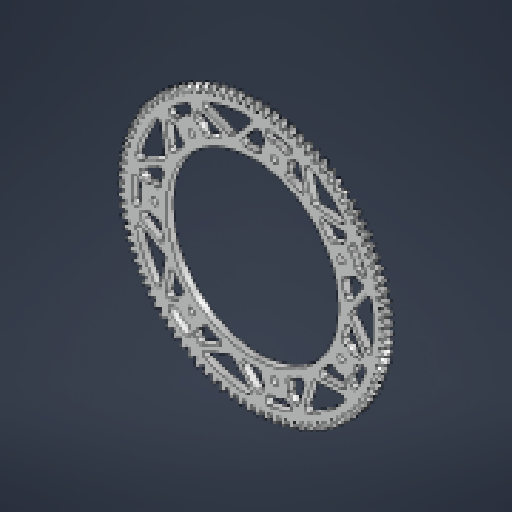
# Autodesk Inventor part: PLATE,TURRET,GEAR
Saved by Autodesk Inventor 2026 (Build 300175000, 175)
## iProperties
CustomPartVersion: 1
Created: 2026-02-09
Part Number: PLATE,TURRET,GEAR
Material: Aluminum 6061
Document SubType Name: Modeling
Designer: littl
Categories: <?xml version="1.0" encoding="UTF-16"?> <MemberInstance><Categories><FamilyTemplate><FamilyTemplateParameter ValueType="xs:double" Id="1" ObjectReferenceKey="da_z" ObjectType="kUserParameterObject"/><FamilyTemplateParameter ValueType="xs:double" Id="2" ObjectReferenceKey="da_b" ObjectType="kUserParameterObject"/><FamilyTemplateParameter ValueType="xs:double" Id="3" ObjectReferenceKey="da_beta" ObjectType="kUserParameterObject"/><FamilyTemplateParameter ValueType="xs:double" Id="4" ObjectReferenceKey="da_da" ObjectType="kUserParameterObject"/><FamilyTemplateParameter ValueType="xs:double" Id="5" ObjectReferenceKey="da_aw" ObjectType="kUserParameterObject"/><FamilyTemplateParameter ValueType="xs:string" Id="6" ObjectReferenceKey="EAIAABAAAAC/AAAAAAAAAIAAAAAAAAAA" ObjectType="83910656" SubObjectId="SurfaceGeometry"/></FamilyTemplate><ParamToTemplateMap><ParamToTemplate CategoryParameter="//CategoryParameter[@InternalName='046C89C9-8512-4d59-83FE-43B91F4F132A']" TemplateParameter="1"/><ParamToTemplate CategoryParameter="//CategoryParameter[@InternalName='2552DF32-E462-4b46-AEBF-C6C7768E72AC']" TemplateParameter="2"/><ParamToTemplate CategoryParameter="//CategoryParameter[@InternalName='C9EE641D-15FC-4fae-A226-E94C4372FDD7']" TemplateParameter="3"/><ParamToTemplate><ParamToTemplate CategoryParameter="//CategoryParameter[@InternalName='00B6519A-459B-49c7-AD84-2E56D39A5744']" ConstantValue="0.000000"/></ParamToTemplate><ParamToTemplate><ParamToTemplate CategoryParameter="//CategoryParameter[@InternalName='04B31F0E-C7A6-4894-AA32-9629BEFACF47']" ConstantValue="1.000000"/></ParamToTemplate><ParamToTemplate><ParamToTemplate CategoryParameter="//CategoryParameter[@InternalName='43CBEC2E-7847-49e7-A936-2F7889FCB2D9']" ConstantValue="0.250000"/></ParamToTemplate><ParamToTemplate><ParamToTemplate CategoryParameter="//CategoryParameter[@InternalName='B1EFC894-105D-4ebd-86BF-FA20ED196853']" ConstantValue="0.350000"/></ParamToTemplate><ParamToTemplate><ParamToTemplate CategoryParameter="//CategoryParameter[@InternalName='51175063-3D10-4879-93E8-6246FE8B403D']" ConstantValue="2061532430.657340"/></ParamToTemplate><ParamToTemplate><ParamToTemplate CategoryParameter="//CategoryParameter[@InternalName='A3A52E27-4454-46a9-B0BD-C932399B70AF']" ConstantValue="0.300000"/></ParamToTemplate><ParamToTemplate><ParamToTemplate CategoryParameter="//CategoryParameter[@InternalName='91B76062-C214-41d9-B1B9-14D2AB99603D']" ConstantValue="0.254000"/></ParamToTemplate><ParamToTemplate><ParamToTemplate CategoryParameter="//CategoryParameter[@InternalName='374E806E-8B8A-4dda-A9AA-1039D6500AD2']" ConstantValue="3.937008"/></ParamToTemplate><ParamToTemplate><ParamToTemplate CategoryParameter="//CategoryParameter[@InternalName='2D373A89-B862-43d6-8D0B-0CBF12AB9F6C']" ConstantValue="0.349066"/></ParamToTemplate><ParamToTemplate CategoryParameter="//CategoryParameter[@InternalName='37777632-D6A2-4fac-9D53-DB8ACD95C989']" TemplateParameter="4"/><ParamToTemplate CategoryParameter="//CategoryParameter[@InternalName='FD1017F1-B727-4f7e-9707-0F86F1FF9423']" TemplateParameter="5"/><ParamToTemplate><ParamToTemplate CategoryParameter="//CategoryParameter[@InternalName='9E1B4470-B2D3-4ff1-B813-535BB4CDF51A']" ConstantValue="3523220.976809"/></ParamToTemplate><ParamToTemplate><ParamToTemplate CategoryParameter="//CategoryParameter[@InternalName='F8452263-BFF6-458c-9FB1-07C4B99E95CD']" ConstantValue="11397033.805607"/></ParamToTemplate><ParamToTemplate><ParamToTemplate CategoryParameter="//CategoryParameter[@InternalName='3E3BB259-FD49-497f-8171-6EBC954A3479']" ConstantValue="2.000000"/></ParamToTemplate><ParamToTemplate CategoryParameter="//CategoryParameter[@InternalName='27C3BAF2-7550-4e4b-AE2C-0DB134B7D9B7']" TemplateParameter="6"/></ParamToTemplateMap><Category DisplayName="Gear" InternalName="DC85795E-93AB-48d5-8EEE-5A27447B64BD" Mnemonic="Gear"><CategoryParameter DisplayName="z" InternalName="046C89C9-8512-4d59-83FE-43B91F4F132A" Mnemonic="z"/><CategoryParameter DisplayName="b" InternalName="2552DF32-E462-4b46-AEBF-C6C7768E72AC" Mnemonic="b"/><CategoryParameter DisplayName="||b|" InternalName="C9EE641D-15FC-4fae-A226-E94C4372FDD7" Mnemonic="beta"/><CategoryParameter DisplayName="x" InternalName="00B6519A-459B-49c7-AD84-2E56D39A5744" Mnemonic="x"/><CategoryParameter DisplayName="a*" InternalName="04B31F0E-C7A6-4894-AA32-9629BEFACF47" Mnemonic="a"/><CategoryParameter DisplayName="c*" InternalName="43CBEC2E-7847-49e7-A936-2F7889FCB2D9" Mnemonic="c"/><CategoryParameter DisplayName="r|.f|*" InternalName="B1EFC894-105D-4ebd-86BF-FA20ED196853" Mnemonic="rf"/><CategoryParameter DisplayName="E" InternalName="51175063-3D10-4879-93E8-6246FE8B403D" Mnemonic="E"/><CategoryParameter DisplayName="||m|" InternalName="A3A52E27-4454-46a9-B0BD-C932399B70AF" Mnemonic="mi"/><Category DisplayName="SpurGear" InternalName="26C5A22E-A91E-4dfd-A3B3-23CCAFAE1764" Mnemonic="SpurGear"><CategoryParameter DisplayName="m" InternalName="91B76062-C214-41d9-B1B9-14D2AB99603D" Mnemonic="m"/><CategoryParameter DisplayName="P" InternalName="374E806E-8B8A-4dda-A9AA-1039D6500AD2" Mnemonic="PP"/><CategoryParameter DisplayName="||a|" InternalName="2D373A89-B862-43d6-8D0B-0CBF12AB9F6C" Mnemonic="alpha"/><CategoryParameter DisplayName="d|.a|" InternalName="37777632-D6A2-4fac-9D53-DB8ACD95C989" Mnemonic="da"/><CategoryParameter DisplayName="a|.w|" InternalName="FD1017F1-B727-4f7e-9707-0F86F1FF9423" Mnemonic="aw"/><CategoryParameter DisplayName="||s||.Flim|" InternalName="9E1B4470-B2D3-4ff1-B813-535BB4CDF51A" Mnemonic="sFlim"/><CategoryParameter DisplayName="||s||.Hlim|" InternalName="F8452263-BFF6-458c-9FB1-07C4B99E95CD" Mnemonic="sHlim"/><CategoryParameter DisplayName="type" InternalName="3E3BB259-FD49-497f-8171-6EBC954A3479" Mnemonic="type"/><CategoryParameter DisplayName="PitchDiameter" InternalName="27C3BAF2-7550-4e4b-AE2C-0DB134B7D9B7" Mnemonic="IDS_PITCHDIAM"/></Category></Category></Categories></MemberInstance>
Density: 2.7 g/cm^3
Appearance: Aluminum - Flat
Mass: 279.635 g
Surface Area: 594.33 cm^2
Volume: 103.568 cm^3
Author: littl
Autodesk Inventor part; units mm, degrees
sketch "Sketch1" plane through (0, 0, 0) normal (0, 0, 1) x (1, 0, 0)
  circle A0 centre (0, 0) radius 123.19
  dimension "d0" = 246.38
  constraints: 1 centre point
  measures "d0" diameter of A0
extrude "Extrusion1" add sketch "Sketch1" along normal blind 6.35
sketch "Sketch2" plane through (0, 0, 0) normal (0, 0, -1) x (-1, 0, 0)
  circle A0 centre (0, 0) radius 123.19 projected
  circle A1 centre (0, 0) radius 120.65
  dimension "d3" = 241.3
  constraints: 1 centre point, 1 coincident
  measures "d3" diameter of A1
surface extrude "Pitch Diameter" sketch "Sketch2" against normal through all shown no curves A1
ref_plane "Work Plane1" through (0, 0, 0) normal (1, 0, 0) x (0, 1, 0)
ref_plane "Work Plane2" through (0, 0, 0) normal (0.9994533, 0.0330634, 0) x (0, 0, 1)
ref_plane "Work Plane3" through (0, 0, 3.175) normal (0, 0, -1) x (-1, 0, 0)
spur gear teeth "Spur Gear" teeth 95 pitch diameter 241.3 tip diameter 246.38 root diameter 234.95 face width 6.35 start plane through (0, 0, 0) normal (0, 0, -1) x (-1, 0, 0)
sketch "Sketch3" plane through (0, 0, 6.35) normal (0, 0, 1) x (1, 0, 0)
  circle A0 centre (0, 0) radius 79.375
  dimension "d20" = 158.75
  constraints: 1 centre point, 1 coincident
  measures "d20" diameter of A0
extrude "Extrusion2" cut sketch "Sketch3" against normal through all
sketch "Sketch4" plane through (0, 0, 6.35) normal (0, 0, 1) x (1, 0, 0)
  point P0 (0, 0)
  point P1 (-90.4875, 0)
  point P2 (-56.418, -70.746)
  point P3 (20.1354, -88.2188)
  point P4 (81.5264, -39.2611)
  point P5 (81.5264, 39.2611)
  point P6 (20.1354, 88.2188)
  point P7 (-56.418, 70.746)
  dimension "d23" = 90.4875
  dimension "d26" = 360
  constraints: 1 horizontal alignment, 8 other
  measures "d23" distance of point (0, 0) point (-90.487, 0)
hole "Hole1" at (-90.4875, 0, 6.35) at (-56.418, -70.746, 6.35) at (20.1354, -88.2188, 6.35) at (81.5264, -39.2611, 6.35) at (81.5264, 39.2611, 6.35) at (20.1354, 88.2188, 6.35) at (-56.418, 70.746, 6.35) direction (0, 0, -1) diameter 6.35 end through all
sketch "Sketch6" plane through (0, 0, 6.35) normal (0, 0, 1) x (1, 0, 0)
  circle A0 centre (-56.418, -70.746) radius 3.175 projected
  circle A1 centre (-56.418, -70.746) radius 12.7
  circle A2 centre (-90.4875, 0) radius 3.175 projected
  circle A3 centre (-90.4875, 0) radius 12.7
  circle A4 centre (-56.418, 70.746) radius 3.175 projected
  circle A5 centre (-56.418, 70.746) radius 12.7
  circle A6 centre (20.1354, 88.2188) radius 3.175 projected
  circle A7 centre (20.1354, 88.2188) radius 12.7
  circle A8 centre (20.1354, -88.2188) radius 3.175 projected
  circle A9 centre (20.1354, -88.2188) radius 12.7
  circle A10 centre (81.5264, -39.2611) radius 3.175 projected
  circle A11 centre (81.5264, -39.2611) radius 12.7
  circle A12 centre (81.5264, 39.2611) radius 3.175 projected
  circle A13 centre (81.5264, 39.2611) radius 12.7
  circle A14 centre (0, 0) radius 85.725
  circle A15 centre (0, 0) radius 111.125
  line L0 (-90.4875, 0) -> (-109.4885, -19.001) construction
  line L1 (-92.1713, 1.6838) -> (-111.1723, -17.3172)
  line L2 (-107.8047, -20.6848) -> (-88.8037, -1.6838)
  arc A16 (-88.8037, -1.6838) -> (-92.1713, 1.6838) centre (-90.4875, 0) ccw
  arc A17 (-111.1723, -17.3172) -> (-107.8047, -20.6848) centre (-109.4885, -19.001) ccw
  line L3 (-90.4875, 0) -> (-63.6161, 0) construction
  line L4 (-90.4875, 0) -> (-109.4885, 19.001) construction
  line L5 (-88.8037, 1.6838) -> (-107.8047, 20.6848)
  line L6 (-111.1723, 17.3172) -> (-92.1713, -1.6838)
  arc A18 (-92.1713, -1.6838) -> (-88.8037, 1.6838) centre (-90.4875, 0) ccw
  arc A19 (-107.8047, 20.6848) -> (-111.1723, 17.3172) centre (-109.4885, 19.001) ccw
  line L7 (-90.4875, 0) -> (-63.6161, 0) construction
  line L8 (-107.8047, -20.6848) -> (-108.9581, -21.8382)
  line L9 (-107.8047, 20.6848) -> (-108.9581, 21.8382)
  line L10 (-58.7843, -71.0126) -> (-55.7757, -97.7151)
  line L11 (-51.0431, -97.1818) -> (-54.0518, -70.4794)
  line L12 (-51.0431, -97.1818) -> (-50.8605, -98.8027)
  line L13 (-56.6846, -68.3797) -> (-83.3871, -71.3883)
  line L14 (-82.8539, -76.1209) -> (-56.1514, -73.1123)
  line L15 (-83.3871, -71.3883) -> (-85.008, -71.571)
  line L16 (18.8685, -90.2351) -> (41.6212, -104.5315)
  line L17 (44.155, -100.499) -> (21.4023, -86.2025)
  line L18 (44.155, -100.499) -> (45.5361, -101.3668)
  line L19 (18.1191, -86.9519) -> (3.8226, -109.7046)
  line L20 (7.8552, -112.2384) -> (22.1516, -89.4857)
  line L21 (3.8226, -109.7046) -> (2.9548, -111.0857)
  line L22 (82.3129, -41.5087) -> (107.6764, -32.6336)
  line L23 (106.1035, -28.1384) -> (80.7399, -37.0134)
  line L24 (106.1035, -28.1384) -> (107.643, -27.5996)
  line L25 (79.2788, -40.0475) -> (88.1539, -65.411)
  line L26 (92.6491, -63.8381) -> (83.774, -38.4746)
  line L27 (88.1539, -65.411) -> (88.6926, -66.9506)
  line L28 (83.774, 38.4746) -> (92.6491, 63.8381)
  line L29 (88.1539, 65.411) -> (79.2788, 40.0475)
  line L30 (88.1539, 65.411) -> (88.6926, 66.9506)
  line L31 (80.7399, 37.0134) -> (106.1035, 28.1384)
  line L32 (107.6764, 32.6336) -> (82.3129, 41.5087)
  line L33 (106.1035, 28.1384) -> (107.643, 27.5996)
  line L34 (22.1516, 89.4857) -> (7.8552, 112.2384)
  line L35 (3.8226, 109.7046) -> (18.1191, 86.9519)
  line L36 (3.8226, 109.7046) -> (2.9548, 111.0857)
  line L37 (21.4023, 86.2025) -> (44.155, 100.499)
  line L38 (41.6212, 104.5315) -> (18.8685, 90.2351)
  line L39 (44.155, 100.499) -> (45.5361, 101.3668)
  line L40 (-56.1514, 73.1123) -> (-82.8539, 76.1209)
  line L41 (-83.3871, 71.3883) -> (-56.6846, 68.3797)
  line L42 (-83.3871, 71.3883) -> (-85.008, 71.571)
  line L43 (-54.0518, 70.4794) -> (-51.0431, 97.1818)
  line L44 (-55.7757, 97.7151) -> (-58.7843, 71.0126)
  line L45 (-51.0431, 97.1818) -> (-50.8605, 98.8027)
  line L46 (-109.4885, -19.001) -> (-77.2356, -37.1947) construction
  line L47 (-110.6584, -21.075) -> (-78.4055, -39.2687)
  line L48 (-76.0656, -35.1207) -> (-108.3185, -16.927)
  arc A20 (-108.3185, -16.927) -> (-110.6584, -21.075) centre (-109.4885, -19.001) ccw
  arc A21 (-78.4055, -39.2687) -> (-76.0656, -35.1207) centre (-77.2356, -37.1947) ccw
  line L49 (-77.2356, -37.1947) -> (-83.1205, -73.7546) construction
  line L50 (-79.5865, -36.8163) -> (-85.4715, -73.3762)
  line L51 (-80.7695, -74.1331) -> (-74.8846, -37.5731)
  arc A22 (-74.8846, -37.5731) -> (-79.5865, -36.8163) centre (-77.2356, -37.1947) ccw
  arc A23 (-85.4715, -73.3762) -> (-80.7695, -74.1331) centre (-83.1205, -73.7546) ccw
  line L52 (-83.1205, -73.7546) -> (-56.418, -70.746) construction
  line L53 (-20.8373, -85.1778) -> (4.0772, -112.5736)
  line L54 (-52.5173, -99.6563) -> (-18.1835, -85.7835)
  line L55 (-19.9677, -81.3679) -> (-54.3015, -95.2406)
  line L56 (7.6006, -109.3694) -> (-17.3139, -81.9736)
  line L57 (53.6029, -69.3988) -> (90.5557, -67.0008)
  line L58 (45.1704, -103.1944) -> (55.731, -67.7016)
  line L59 (51.1663, -66.3434) -> (40.6057, -101.8362)
  line L60 (90.2473, -62.2483) -> (53.2945, -64.6463)
  line L61 (87.679, -1.361) -> (108.8439, 29.025)
  line L62 (108.8439, -29.025) -> (87.679, 1.361)
  line L63 (83.771, -1.361) -> (104.936, -31.747)
  line L64 (104.936, 31.747) -> (83.771, 1.361)
  line L65 (55.731, 67.7016) -> (45.1704, 103.1944)
  line L66 (90.5557, 67.0008) -> (53.6029, 69.3988)
  line L67 (53.2945, 64.6463) -> (90.2473, 62.2483)
  line L68 (40.6057, 101.8362) -> (51.1663, 66.3434)
  line L69 (-18.1835, 85.7835) -> (-52.5173, 99.6563)
  line L70 (4.0772, 112.5736) -> (-20.8373, 85.1778)
  line L71 (-17.3139, 81.9736) -> (7.6006, 109.3694)
  line L72 (-54.3015, 95.2406) -> (-19.9677, 81.3679)
  line L73 (-78.4055, 39.2687) -> (-110.6584, 21.075)
  line L74 (-85.4715, 73.3762) -> (-79.5865, 36.8163)
  line L75 (-74.8846, 37.5731) -> (-80.7695, 74.1331)
  line L76 (-108.3185, 16.927) -> (-76.0656, 35.1207)
  point P0 (-99.988, -9.5005)
  point P1 (-99.988, 9.5005)
  point P2 (-93.362, -28.0978)
  point P3 (-80.178, -55.4747)
  point P4 (-100.9923, 7.1372)
  point P5 (-109.9528, 16.0977)
  point P6 (-109.9528, -16.0977)
  point P7 (-100.9923, -7.1372)
  point P8 (-75.4015, -40.7846)
  point P9 (-80.2712, -71.0373)
  point P10 (-69.081, -69.7764)
  point P11 (-61.9103, -59.295)
  point P12 (-99.6769, -73.2238)
  point P13 (-79.8501, -38.4538)
  point P14 (-119.3962, -32.2763)
  point P15 (-85.008, -71.571)
  point P16 (-105.5875, -18.4675)
  point P17 (-78.8988, -33.5225)
  point P18 (-84.9591, -11.4336)
  point P19 (-97.6247, -10.5048)
  point P20 (-78.8988, 33.5225)
  point P21 (-105.5875, 18.4675)
  point P22 (-97.6247, 10.5048)
  point P23 (-84.9591, 11.4336)
  point P24 (-80.2712, 71.0373)
  point P25 (-75.4015, 40.7846)
  point P26 (-61.9103, 59.295)
  point P27 (-69.081, 69.7764)
  point P28 (-79.8501, 38.4538)
  point P29 (-99.6769, 73.2238)
  point P30 (-85.008, 71.571)
  point P31 (-119.3962, 32.2763)
  point P32 (-57.3876, 83.4089)
  point P33 (-55.9688, 96.0014)
  point P34 (-81.1402, 75.9278)
  point P35 (-68.5477, 74.509)
  point P36 (-22.9837, 82.5865)
  point P37 (-51.3942, 94.0659)
  point P38 (-52.655, 82.8757)
  point P39 (-44.032, 73.5524)
  point P40 (-19.7214, 86.4049)
  point P41 (-4.8989, 123.5848)
  point P42 (2.9548, 111.0857)
  point P43 (-50.8605, 98.8027)
  point P44 (-49.2077, 113.4716)
  point P45 (5.4909, 107.0496)
  point P46 (-15.1254, 84.3801)
  point P47 (7.7583, 85.3732)
  point P48 (11.4821, 97.5146)
  point P49 (29.4311, 96.872)
  point P50 (40.161, 103.614)
  point P51 (8.7727, 110.7782)
  point P52 (15.5147, 100.0484)
  point P53 (50.2386, 69.4612)
  point P54 (41.4999, 98.8307)
  point P55 (31.9649, 92.8395)
  point P56 (30.0521, 80.2848)
  point P57 (55.258, 69.2914)
  point P58 (93.5681, 80.884)
  point P59 (45.5361, 101.3668)
  point P60 (58.0352, 109.2205)
  point P61 (87.1182, 62.4514)
  point P62 (56.5405, 64.4356)
  point P63 (71.5847, 47.1637)
  point P64 (83.399, 51.8223)
  point P65 (94.0876, 37.3885)
  point P66 (106.0486, 33.2032)
  point P67 (92.0795, 62.2103)
  point P68 (87.8942, 50.2493)
  point P69 (88.627, 0)
  point P70 (121.5764, -22.7241)
  point P71 (107.643, -27.5996)
  point P72 (107.643, 27.5996)
  point P73 (121.5764, 22.7241)
  point P74 (85.6302, 4.0302)
  point P75 (103.1438, 29.174)
  point P76 (92.5147, 32.8933)
  point P77 (81.5064, 26.5611)
  point P78 (103.1438, -29.174)
  point P79 (85.6302, -4.0302)
  point P80 (81.5064, -26.5611)
  point P81 (92.5147, -32.8933)
  point P82 (87.8942, -50.2493)
  point P83 (92.0795, -62.2103)
  point P84 (106.0486, -33.2032)
  point P85 (94.0876, -37.3885)
  point P86 (56.5405, -64.4356)
  point P87 (87.1182, -62.4514)
  point P88 (83.399, -51.8223)
  point P89 (71.5847, -47.1637)
  point P90 (55.258, -69.2914)
  point P91 (58.0352, -109.2205)
  point P92 (45.5361, -101.3668)
  point P93 (88.6926, -66.9506)
  point P94 (93.5681, -80.884)
  point P95 (41.4999, -98.8307)
  point P96 (50.2386, -69.4612)
  point P97 (30.0521, -80.2848)
  point P98 (31.9649, -92.8395)
  point P99 (15.5147, -100.0484)
  point P100 (8.7727, -110.7782)
  point P101 (40.161, -103.614)
  point P102 (29.4311, -96.872)
  point P103 (-15.1254, -84.3801)
  point P104 (5.4909, -107.0496)
  point P105 (11.4821, -97.5146)
  point P106 (7.7583, -85.3732)
  point P107 (-19.7214, -86.4049)
  point P108 (-49.2077, -113.4716)
  point P109 (-50.8605, -98.8027)
  point P110 (2.9548, -111.0857)
  point P111 (-4.8989, -123.5848)
  point P112 (-51.3942, -94.0659)
  point P113 (-22.9837, -82.5865)
  point P114 (-44.032, -73.5524)
  point P115 (-52.655, -82.8757)
  point P116 (-68.5477, -74.509)
  point P117 (-81.1402, -75.9278)
  point P118 (-55.9688, -96.0014)
  point P119 (-57.3876, -83.4089)
  point P120 (-85.1531, -71.3983)
  point P121 (-109.8705, -16.6506)
  point P122 (-108.9135, -22.0593)
  point P123 (-81.5211, -75.5187)
  point P124 (-85.1531, 71.3983)
  point P125 (-108.9135, 22.0593)
  point P126 (2.7293, 111.0915)
  point P127 (-50.6598, 98.9058)
  point P128 (88.5565, 67.1306)
  point P129 (45.7418, 101.2742)
  point P130 (107.6989, -27.381)
  point P131 (107.6989, 27.381)
  point P132 (45.7418, -101.2742)
  point P133 (88.5565, -67.1306)
  point P134 (-50.6598, -98.9058)
  point P135 (2.7293, -111.0915)
  dimension "d51" = 171.45
  dimension "d52" = 222.25
  dimension "d50" = 25.4
  dimension "d53" = 135
  dimension "d54" = 4.7625
  dimension "d55" = 135
  dimension "d56" = 4.7625
  dimension "d59" = 360
  dimension "d61" = 4.7625
  dimension "d62" = 4.7625
  dimension "d65" = 360
  constraints: 162 end point, 16 point on circle, 16 tangent, 15 centre point, 9 coincident, 6 equal radius, 5 parallel, 4 midpoint, 3 equal length, 2 collinear, 2 horizontal, 208 other
  measures "d50" diameter of A1
  measures "d53" angle of L0 L3
  measures "d54" diameter of A17
  measures "d55" angle of L7 L4
  measures "d56" diameter of A19
  measures "d61" diameter of A21
  measures "d62" diameter of A23
extrude "Extrusion4" cut sketch "Sketch6" against normal through all contours L13 L51 A14 A1 | A1 A14 L55 L11 | A1 L10 A15 L14 | A14 A9 L19 L56 | A15 L47 L50 | L54 L53 A15 | L48 L2 A3 A14 | A14 L59 L17 A9 | A9 L16 A15 L20 | A3 L5 L76 A14 | A14 A11 L25 L60 | L1 A15 L6 A3 | L75 L41 A5 A14 | A14 L63 L23 A11 | L58 L57 A15 | A11 L22 A15 L26 | A5 L43 L72 A14 | A15 L74 L73 | L40 A15 L44 A5 | A14 A13 L31 L64 | L71 L35 A7 A14 | L62 L61 A15 | A14 L67 L29 A13 | A7 L37 L68 A14 | A13 L28 A15 L32 | A15 L70 L69 | L34 A15 L38 A7 | L66 L65 A15
fillet "Fillet4" radius 3.175 15 edges at (-75.4015, 40.7846, 3.175) (-79.8501, 38.4538, 3.175) (-61.9103, 59.295, 3.175) (-69.081, 69.7764, 3.175) (-80.2712, 71.0373, 3.175) (-81.1402, 75.9278, 3.175) (-68.5477, 74.509, 3.175) (-57.3876, 83.4089, 3.175) (-55.9688, 96.0014, 3.175) (-51.3942, 94.0659, 3.175) (-52.655, 82.8757, 3.175) (-44.032, 73.5524, 3.175) (-22.9837, 82.5865, 3.175) (-85.1531, 71.3983, 3.175) (-50.6598, 98.9058, 3.175)
pattern_circular "Circular Pattern1" count 7 over 360 about axis through (0, 0, 0) along (0, 0, -1) of "Fillet4"
equation "\"d0\" = da_da"
equation "\"d1\" = da_b"
equation "\"d3\" = da_d"
equation "\"d15\" = da_aw"
equation "\"d19\" = da_aw"
equation "\"da_da\" = 246.38"
equation "\"da_b\" = 6.35"
equation "\"da_d\" = 241.3"
equation "\"da_aw\" = 241.3"
body "Solid1"
body "Srf1"
